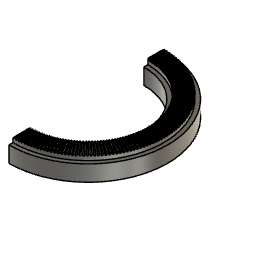
Angled Rack and BEVEL track system - Light output v2 (Autodesk Fusion 360 design; units mm, degrees)
Autodesk Fusion 360 part; units mm, degrees
sketch "Sketch1" plane through (0, 0, 0) normal (0, 0, 1) x (1, 0, 0)
  circle A0 centre (0, 0) radius 100
  dimension "d1" = 200
  constraint coincident A0.centre origin
  measures "d1" diameter of A0
sketch "Sketch2" plane through (0, 0, 0) normal (0, 0, 1) x (1, 0, 0)
  circle A0 centre (0, 0) radius 100
  line L0 (0, 100) -> (0, -100)
  constraint coincident A0 L0.start
  constraint coincident A0 L0.end
  constraint vertical L0
extrude "Extrude1" add sketch "Sketch2" along normal blind 20 contours A0 L0 picked at (53.8118, -17.5328)
sketch "Sketch3" plane through (0, 0, 20) normal (0, 0, 1) x (-1, 0, 0)
  line L0 (0, -100) -> (0, 100)
  arc A0 (0, 100) -> (0, -100) centre (0, 0) ccw
  circle A1 centre (0, 0) radius 70
  dimension "d4" = 140
  constraint coincident A0.centre A1.centre
  measures "d4" diameter of A1
extrude "Extrude2" cut sketch "Sketch3" against normal blind 30 contours L0 A1 picked at (-23.2681, 1.7437)
sketch "Sketch4" plane through (0, 0, 20) normal (0, 0, 1) x (-1, 0, 0)
  arc A0 (0, 70) -> (0, -70) centre (0, 0) ccw
  line L0 (0, 70) -> (0, 100)
  arc A1 (0, 100) -> (0, -100) centre (0, 0) ccw
  line L1 (0, -100) -> (0, -70)
  circle A2 centre (0, 0) radius 75
  circle A3 centre (0, 0) radius 95
  dimension "d7" = 150
  dimension "d8" = 190
  constraint coincident A0.centre A1.centre
  measures "d7" diameter of A2
  measures "d8" diameter of A3
extrude "Extrude3" add sketch "Sketch4" along normal blind 5 contours L0 L1 A2 A3 picked at (-4.7197, -87.9796)
sketch "Sketch5" plane through (0, 0, 25) normal (0, 0, 1) x (-1, 0, 0)
  line L0 (0, 75) -> (0, 95)
  arc A0 (0, 95) -> (0, -95) centre (0, 0) ccw
  line L1 (0, -95) -> (0, -75)
  arc A1 (0, 75) -> (0, -75) centre (0, 0) ccw
  line L2 (0, 0) -> (0, -95)
  line L3 (0, 0) -> (-1.658, -94.9855)
  line L4 (0, 0) -> (95, 0) construction
  line L5 (0, 0) -> (-3.3155, -94.9421)
  line L6 (0, 0) -> (95, 0) construction
  line L7 (0, 0) -> (-4.9719, -94.8698)
  line L8 (0, 0) -> (95, 0) construction
  line L9 (0, 0) -> (-6.6269, -94.7686)
  line L10 (0, 0) -> (95, 0) construction
  line L11 (0, 0) -> (-8.2798, -94.6385)
  line L12 (0, 0) -> (95, 0) construction
  line L13 (0, 0) -> (-9.9302, -94.4796)
  line L14 (0, 0) -> (95, 0) construction
  line L15 (0, 0) -> (-11.5776, -94.2919)
  line L16 (0, 0) -> (95, 0) construction
  line L17 (0, 0) -> (-13.2214, -94.0755)
  line L18 (0, 0) -> (95, 0) construction
  line L19 (0, 0) -> (-14.8613, -93.8304)
  line L20 (0, 0) -> (95, 0) construction
  line L21 (0, 0) -> (-16.4966, -93.5567)
  line L22 (0, 0) -> (95, 0) construction
  line L23 (0, 0) -> (-18.1269, -93.2546)
  line L24 (0, 0) -> (95, 0) construction
  line L25 (0, 0) -> (-19.7516, -92.924)
  line L26 (0, 0) -> (95, 0) construction
  line L27 (0, 0) -> (-21.3704, -92.5652)
  line L28 (0, 0) -> (95, 0) construction
  line L29 (0, 0) -> (-22.9826, -92.1781)
  line L30 (0, 0) -> (95, 0) construction
  line L31 (0, 0) -> (-24.5878, -91.763)
  line L32 (0, 0) -> (95, 0) construction
  line L33 (0, 0) -> (-26.1855, -91.3199)
  line L34 (0, 0) -> (95, 0) construction
  line L35 (0, 0) -> (-27.7753, -90.849)
  line L36 (0, 0) -> (95, 0) construction
  line L37 (0, 0) -> (-29.3566, -90.3504)
  line L38 (0, 0) -> (95, 0) construction
  line L39 (0, 0) -> (-30.929, -89.8243)
  line L40 (0, 0) -> (95, 0) construction
  line L41 (0, 0) -> (-32.4919, -89.2708)
  line L42 (0, 0) -> (95, 0) construction
  line L43 (0, 0) -> (-34.045, -88.6901)
  line L44 (0, 0) -> (95, 0) construction
  line L45 (0, 0) -> (-35.5876, -88.0825)
  line L46 (0, 0) -> (95, 0) construction
  line L47 (0, 0) -> (-37.1195, -87.448)
  line L48 (0, 0) -> (95, 0) construction
  line L49 (0, 0) -> (-38.64, -86.7868)
  line L50 (0, 0) -> (95, 0) construction
  line L51 (0, 0) -> (-40.1487, -86.0992)
  line L52 (0, 0) -> (95, 0) construction
  line L53 (0, 0) -> (-41.6453, -85.3854)
  line L54 (0, 0) -> (95, 0) construction
  line L55 (0, 0) -> (-43.1291, -84.6456)
  line L56 (0, 0) -> (95, 0) construction
  line L57 (0, 0) -> (-44.5998, -83.88)
  line L58 (0, 0) -> (95, 0) construction
  line L59 (0, 0) -> (-46.0569, -83.0889)
  line L60 (0, 0) -> (95, 0) construction
  line L61 (0, 0) -> (-47.5, -82.2724)
  line L62 (0, 0) -> (95, 0) construction
  line L63 (0, 0) -> (-48.9286, -81.4309)
  line L64 (0, 0) -> (95, 0) construction
  line L65 (0, 0) -> (-50.3423, -80.5646)
  line L66 (0, 0) -> (95, 0) construction
  line L67 (0, 0) -> (-51.7407, -79.6737)
  line L68 (0, 0) -> (95, 0) construction
  line L69 (0, 0) -> (-53.1233, -78.7586)
  line L70 (0, 0) -> (95, 0) construction
  line L71 (0, 0) -> (-54.4898, -77.8194)
  line L72 (0, 0) -> (95, 0) construction
  line L73 (0, 0) -> (-55.8396, -76.8566)
  line L74 (0, 0) -> (95, 0) construction
  line L75 (0, 0) -> (0, -2.1876)
  line L76 (0, 0) -> (-57.1724, -75.8704)
  line L77 (0, 0) -> (95, 0) construction
  line L78 (0, 0) -> (-58.4878, -74.861)
  line L79 (0, 0) -> (95, 0) construction
  line L80 (0, 0) -> (-59.7854, -73.8289)
  line L81 (0, 0) -> (95, 0) construction
  line L82 (0, 0) -> (-61.0648, -72.7742)
  line L83 (0, 0) -> (95, 0) construction
  line L84 (0, 0) -> (-62.3256, -71.6974)
  line L85 (0, 0) -> (95, 0) construction
  line L86 (0, 0) -> (-63.5674, -70.5988)
  line L87 (0, 0) -> (95, 0) construction
  line L88 (0, 0) -> (-64.7898, -69.4786)
  line L89 (0, 0) -> (95, 0) construction
  line L90 (0, 0) -> (-65.9925, -68.3373)
  line L91 (0, 0) -> (95, 0) construction
  line L92 (0, 0) -> (-67.1751, -67.1751)
  line L93 (0, 0) -> (95, 0) construction
  line L94 (0, 0) -> (-68.3373, -65.9925)
  line L95 (0, 0) -> (95, 0) construction
  line L96 (0, 0) -> (-69.4786, -64.7898)
  line L97 (0, 0) -> (95, 0) construction
  line L98 (0, 0) -> (-70.5988, -63.5674)
  line L99 (0, 0) -> (95, 0) construction
  line L100 (0, 0) -> (-71.6974, -62.3256)
  line L101 (0, 0) -> (95, 0) construction
  line L102 (0, 0) -> (-72.7742, -61.0648)
  line L103 (0, 0) -> (95, 0) construction
  line L104 (0, 0) -> (-73.8289, -59.7854)
  line L105 (0, 0) -> (95, 0) construction
  line L106 (0, 0) -> (-74.861, -58.4878)
  line L107 (0, 0) -> (95, 0) construction
  line L108 (0, 0) -> (-75.8704, -57.1724)
  line L109 (0, 0) -> (95, 0) construction
  line L110 (0, 0) -> (-76.8566, -55.8396)
  line L111 (0, 0) -> (95, 0) construction
  line L112 (0, 0) -> (-77.8194, -54.4898)
  line L113 (0, 0) -> (95, 0) construction
  line L114 (0, 0) -> (-78.7586, -53.1233)
  line L115 (0, 0) -> (95, 0) construction
  line L116 (0, 0) -> (-79.6737, -51.7407)
  line L117 (0, 0) -> (95, 0) construction
  line L118 (0, 0) -> (-80.5646, -50.3423)
  line L119 (0, 0) -> (95, 0) construction
  line L120 (0, 0) -> (-81.4309, -48.9286)
  line L121 (0, 0) -> (95, 0) construction
  line L122 (0, 0) -> (-82.2724, -47.5)
  line L123 (0, 0) -> (95, 0) construction
  line L124 (0, 0) -> (-83.0889, -46.0569)
  line L125 (0, 0) -> (95, 0) construction
  line L126 (0, 0) -> (-83.88, -44.5998)
  line L127 (0, 0) -> (95, 0) construction
  line L128 (0, 0) -> (-84.6456, -43.1291)
  line L129 (0, 0) -> (95, 0) construction
  line L130 (0, 0) -> (-85.3854, -41.6453)
  line L131 (0, 0) -> (95, 0) construction
  line L132 (0, 0) -> (94.9855, 0) construction
  line L133 (0, 0) -> (-86.7868, -38.64)
  line L134 (0, 0) -> (95, 0) construction
  line L135 (0, 0) -> (-87.448, -37.1195)
  line L136 (0, 0) -> (95, 0) construction
  line L137 (0, 0) -> (-88.0825, -35.5876)
  line L138 (0, 0) -> (95, 0) construction
  line L139 (0, 0) -> (-88.6901, -34.045)
  line L140 (0, 0) -> (95, 0) construction
  line L141 (0, 0) -> (-89.2708, -32.4919)
  line L142 (0, 0) -> (95, 0) construction
  line L143 (0, 0) -> (-89.8243, -30.929)
  line L144 (0, 0) -> (95, 0) construction
  line L145 (0, 0) -> (-90.3504, -29.3566)
  line L146 (0, 0) -> (95, 0) construction
  line L147 (0, 0) -> (-90.849, -27.7753)
  line L148 (0, 0) -> (95, 0) construction
  line L149 (0, 0) -> (-91.3199, -26.1855)
  line L150 (0, 0) -> (95, 0) construction
  line L151 (0, 0) -> (-91.763, -24.5878)
  line L152 (0, 0) -> (95, 0) construction
  line L153 (0, 0) -> (-92.1781, -22.9826)
  line L154 (0, 0) -> (95, 0) construction
  line L155 (0, 0) -> (-92.5652, -21.3704)
  line L156 (0, 0) -> (95, 0) construction
  line L157 (0, 0) -> (-92.924, -19.7516)
  line L158 (0, 0) -> (95, 0) construction
  line L159 (0, 0) -> (-93.2546, -18.1269)
  line L160 (0, 0) -> (95, 0) construction
  line L161 (0, 0) -> (-93.5567, -16.4966)
  line L162 (0, 0) -> (95, 0) construction
  line L163 (0, 0) -> (-93.8304, -14.8613)
  line L164 (0, 0) -> (95, 0) construction
  line L165 (0, 0) -> (-94.0755, -13.2214)
  line L166 (0, 0) -> (95, 0) construction
  line L167 (0, 0) -> (-94.2919, -11.5776)
  line L168 (0, 0) -> (95, 0) construction
  line L169 (0, 0) -> (-94.4796, -9.9302)
  line L170 (0, 0) -> (95, 0) construction
  line L171 (0, 0) -> (-94.6385, -8.2798)
  line L172 (0, 0) -> (95, 0) construction
  line L173 (0, 0) -> (-94.7686, -6.6269)
  line L174 (0, 0) -> (95, 0) construction
  line L175 (0, 0) -> (-94.8698, -4.9719)
  line L176 (0, 0) -> (95, 0) construction
  line L177 (0, 0) -> (-94.9421, -3.3155)
  line L178 (0, 0) -> (95, 0) construction
  line L179 (0, 0) -> (-94.9855, -1.658)
  line L180 (0, 0) -> (95, 0) construction
  line L181 (0, 0) -> (-95, 0)
  line L182 (0, 0) -> (-86.0992, -40.1487)
  line L183 (0, 0) -> (95, 0) construction
  dimension "d11" = 91
  dimension "d13" = 92
  dimension "d15" = 93
  dimension "d16" = 94
  dimension "d17" = 95
  dimension "d18" = 96
  dimension "d19" = 97
  dimension "d20" = 98
  dimension "d21" = 99
  dimension "d22" = 100
  dimension "d23" = 101
  dimension "d24" = 102
  dimension "d25" = 103
  dimension "d26" = 104
  dimension "d27" = 105
  dimension "d28" = 106
  dimension "d29" = 107
  dimension "d30" = 108
  dimension "d31" = 109
  dimension "d32" = 110
  dimension "d33" = 111
  dimension "d34" = 112
  dimension "d35" = 113
  dimension "d36" = 114
  dimension "d37" = 115
  dimension "d38" = 116
  dimension "d39" = 117
  dimension "d40" = 118
  dimension "d42" = 119
  dimension "d43" = 120
  dimension "d44" = 121
  dimension "d45" = 122
  dimension "d47" = 123
  dimension "d48" = 124
  dimension "d49" = 125
  dimension "d50" = 126
  dimension "d51" = 127
  dimension "d52" = 128
  dimension "d53" = 129
  dimension "d54" = 130
  dimension "d55" = 131
  dimension "d56" = 132
  dimension "d57" = 133
  dimension "d58" = 134
  dimension "d60" = 135
  dimension "d61" = 136
  dimension "d62" = 137
  dimension "d63" = 138
  dimension "d64" = 139
  dimension "d65" = 140
  dimension "d66" = 141
  dimension "d67" = 142
  dimension "d69" = 143
  dimension "d70" = 144
  dimension "d71" = 145
  dimension "d72" = 146
  dimension "d74" = 147
  dimension "d75" = 148
  dimension "d76" = 149
  dimension "d77" = 150
  dimension "d78" = 151
  dimension "d79" = 152
  dimension "d80" = 153
  dimension "d81" = 154
  dimension "d83" = 156
  dimension "d84" = 157
  dimension "d85" = 158
  dimension "d86" = 159
  dimension "d87" = 160
  dimension "d88" = 161
  dimension "d90" = 162
  dimension "d91" = 163
  dimension "d92" = 164
  dimension "d93" = 165
  dimension "d94" = 166
  dimension "d95" = 167
  dimension "d96" = 168
  dimension "d97" = 169
  dimension "d98" = 170
  dimension "d99" = 171
  dimension "d100" = 172
  dimension "d101" = 173
  dimension "d102" = 174
  dimension "d103" = 175
  dimension "d104" = 176
  dimension "d106" = 177
  dimension "d108" = 178
  dimension "d110" = 179
  dimension "d111" = 155
  constraint coincident A0.centre A1.centre
  constraint coincident A0.end L1.start
  constraint horizontal L4
  constraint horizontal L6
  constraint horizontal L8
  constraint horizontal L10
  constraint horizontal L12
  constraint horizontal L14
  constraint horizontal L16
  constraint horizontal L18
  constraint horizontal L20
  constraint horizontal L22
  constraint horizontal L24
  constraint horizontal L26
  constraint horizontal L28
  constraint horizontal L30
  constraint horizontal L32
  constraint horizontal L34
  constraint horizontal L36
  constraint horizontal L38
  constraint horizontal L40
  constraint horizontal L42
  constraint horizontal L44
  constraint horizontal L46
  constraint horizontal L48
  constraint horizontal L50
  constraint horizontal L52
  constraint horizontal L54
  constraint horizontal L56
  constraint horizontal L58
  constraint horizontal L60
  constraint horizontal L62
  constraint horizontal L64
  constraint horizontal L66
  constraint horizontal L68
  constraint horizontal L70
  constraint horizontal L72
  constraint horizontal L74
  constraint vertical L75
  constraint horizontal L77
  constraint horizontal L79
  constraint horizontal L81
  constraint horizontal L83
  constraint horizontal L85
  constraint horizontal L87
  constraint horizontal L89
  constraint horizontal L91
  constraint horizontal L93
  constraint horizontal L95
  constraint horizontal L97
  constraint horizontal L99
  constraint horizontal L101
  constraint horizontal L103
  constraint horizontal L105
  constraint horizontal L107
  constraint horizontal L109
  constraint horizontal L111
  constraint horizontal L113
  constraint horizontal L115
  constraint horizontal L117
  constraint horizontal L119
  constraint horizontal L121
  constraint horizontal L123
  constraint horizontal L125
  constraint horizontal L127
  constraint horizontal L129
  constraint horizontal L131
  constraint horizontal L132
  constraint horizontal L134
  constraint horizontal L136
  constraint horizontal L138
  constraint horizontal L140
  constraint horizontal L142
  constraint horizontal L144
  constraint horizontal L146
  constraint horizontal L148
  constraint horizontal L150
  constraint horizontal L152
  constraint horizontal L154
  constraint horizontal L156
  constraint horizontal L158
  constraint horizontal L160
  constraint horizontal L162
  constraint horizontal L164
  constraint horizontal L166
  constraint horizontal L168
  constraint horizontal L170
  constraint horizontal L172
  constraint horizontal L174
  constraint horizontal L176
  constraint horizontal L178
  constraint horizontal L180
  constraint midpoint A0 L181.end
  constraint horizontal L183
  measures "d11" angle of L3 L4
  measures "d13" angle of L5 L6
  measures "d15" angle of L7 L8
  measures "d16" angle of L9 L10
  measures "d17" angle of L11 L12
  measures "d18" angle of L13 L14
  measures "d19" angle of L15 L16
  measures "d20" angle of L17 L18
  measures "d21" angle of L19 L20
  measures "d22" angle of L21 L22
  measures "d23" angle of L23 L24
  measures "d24" angle of L25 L26
  measures "d25" angle of L27 L28
  measures "d26" angle of L29 L30
  measures "d27" angle of L31 L32
  measures "d28" angle of L33 L34
  measures "d29" angle of L35 L36
  measures "d30" angle of L37 L38
  measures "d31" angle of L39 L40
  measures "d32" angle of L41 L42
  measures "d33" angle of L43 L44
  measures "d34" angle of L45 L46
  measures "d35" angle of L47 L48
  measures "d36" angle of L49 L50
  measures "d37" angle of L51 L52
  measures "d38" angle of L53 L54
  measures "d39" angle of L55 L56
  measures "d40" angle of L57 L58
  measures "d42" angle of L59 L60
  measures "d43" angle of L61 L62
  measures "d44" angle of L63 L64
  measures "d45" angle of L65 L66
  measures "d47" angle of L67 L68
  measures "d48" angle of L69 L70
  measures "d49" angle of L71 L72
  measures "d50" angle of L73 L74
  measures "d51" angle of L76 L77
  measures "d52" angle of L78 L79
  measures "d53" angle of L80 L81
  measures "d54" angle of L82 L83
  measures "d55" angle of L84 L85
  measures "d56" angle of L86 L87
  measures "d57" angle of L88 L89
  measures "d58" angle of L90 L91
  measures "d60" angle of L92 L93
  measures "d61" angle of L94 L95
  measures "d62" angle of L96 L97
  measures "d63" angle of L98 L99
  measures "d64" angle of L100 L101
  measures "d65" angle of L102 L103
  measures "d66" angle of L104 L105
  measures "d67" angle of L106 L107
  measures "d69" angle of L108 L109
  measures "d70" angle of L110 L111
  measures "d71" angle of L112 L113
  measures "d72" angle of L114 L115
  measures "d74" angle of L116 L117
  measures "d75" angle of L118 L119
  measures "d76" angle of L120 L121
  measures "d77" angle of L122 L123
  measures "d78" angle of L124 L125
  measures "d79" angle of L126 L127
  measures "d80" angle of L128 L129
  measures "d81" angle of L130 L131
  measures "d83" angle of L133 L134
  measures "d84" angle of L135 L136
  measures "d85" angle of L137 L138
  measures "d86" angle of L139 L140
  measures "d87" angle of L141 L142
  measures "d88" angle of L143 L144
  measures "d90" angle of L145 L146
  measures "d91" angle of L147 L148
  measures "d92" angle of L149 L150
  measures "d93" angle of L151 L152
  measures "d94" angle of L153 L154
  measures "d95" angle of L155 L156
  measures "d96" angle of L157 L158
  measures "d97" angle of L159 L160
  measures "d98" angle of L161 L162
  measures "d99" angle of L163 L164
  measures "d100" angle of L165 L166
  measures "d101" angle of L167 L168
  measures "d102" angle of L169 L170
  measures "d103" angle of L171 L172
  measures "d104" angle of L173 L174
  measures "d106" angle of L175 L176
  measures "d108" angle of L177 L178
  measures "d110" angle of L179 L180
  measures "d111" angle of L182 L183
sketch "Sketch6" plane through (0, 0, 25) normal (0, 0, 1) x (-1, 0, 0)
sketch "Sketch7" plane through (0, 0, 25) normal (0, 0, 1) x (-1, 0, 0)
sketch "Sketch8" plane through (0, 0, 25) normal (0, 0, 1) x (-1, 0, 0)
extrude "Extrude4" add sketch "Sketch5" along normal blind 2 contours A0 A1 L177 L179 | A0 L1 A1 L2 L3 | A0 A1 L5 L7 | A0 A1 L9 L11 | A0 A1 L13 L15 | A0 A1 L17 L19 | A0 A1 L21 L23 | A0 A1 L25 L27 | A0 A1 L29 L31 | A0 A1 L33 L35 | A0 A1 L37 L39 | A0 A1 L41 L43 | A0 A1 L45 L47 | A0 A1 L49 L51 | A0 A1 L53 L55 | A0 A1 L57 L59 | A0 A1 L61 L63 | A0 A1 L65 L67 | A0 A1 L69 L71 | A0 A1 L73 L76 | A0 A1 L78 L80 | A0 A1 L82 L84 | A0 A1 L86 L88 | A0 A1 L90 L92 | A0 A1 L94 L96 | A0 A1 L98 L100 | A0 A1 L102 L104 | A0 A1 L106 L108 | A0 A1 L110 L112 | A0 A1 L114 L116 | A0 A1 L118 L120 | A0 A1 L122 L124 | A0 A1 L126 L128 | A0 A1 L130 L182 | A0 A1 L133 L135 | A0 A1 L137 L139 | A0 A1 L141 L143 | A0 A1 L145 L147 | A0 A1 L149 L151 | A0 A1 L153 L155 | A0 A1 L157 L159 | A0 A1 L161 L163 | A0 A1 L165 L167 | A0 A1 L169 L171 | A0 A1 L173 L175
sketch "Sketch9" plane through (0, 0, 25) normal (0, 0, 1) x (-1, 0, 0)
  line L0 (-94.9855, -1.658) -> (-74.9886, -1.3089)
  arc A0 (0, 75) -> (-74.9886, -1.3089) centre (0, 0) ccw
  line L1 (0, 75) -> (0, 95)
  arc A1 (0, 95) -> (-94.9855, -1.658) centre (0, 0) ccw
  line L2 (0, 0) -> (-95, 0)
  line L3 (0, 0) -> (-94.9855, 1.658)
  line L4 (0, 0) -> (95, 0) construction
  line L5 (0, 0) -> (-94.9421, 3.3155)
  line L6 (0, 0) -> (95, 0) construction
  line L7 (0, 0) -> (-94.8698, 4.9719)
  line L8 (0, 0) -> (95, 0) construction
  line L9 (0, 0) -> (94.9855, 0) construction
  line L10 (0, 0) -> (94.9855, 0) construction
  line L11 (0, 0) -> (-94.4796, 9.9302)
  line L12 (0, 0) -> (95, 0) construction
  line L13 (0, 0) -> (-94.2919, 11.5776)
  line L14 (0, 0) -> (95, 0) construction
  line L15 (0, 0) -> (-94.0755, 13.2214)
  line L16 (0, 0) -> (94.9421, 0) construction
  line L17 (0, 0) -> (-93.8304, 14.8613)
  line L18 (0, 0) -> (95, 0) construction
  line L19 (0, 0) -> (-93.5567, 16.4966)
  line L20 (0, 0) -> (95, 0) construction
  line L21 (0, 0) -> (-93.2546, 18.1269)
  line L22 (0, 0) -> (95, 0) construction
  line L23 (0, 0) -> (-92.924, 19.7516)
  line L24 (0, 0) -> (95, 0) construction
  line L25 (0, 0) -> (-92.5652, 21.3704)
  line L26 (0, 0) -> (95, 0) construction
  line L27 (0, 0) -> (-92.1781, 22.9826)
  line L28 (0, 0) -> (95, 0) construction
  line L29 (0, 0) -> (-91.763, 24.5878)
  line L30 (0, 0) -> (95, 0) construction
  line L31 (0, 0) -> (-91.3199, 26.1855)
  line L32 (0, 0) -> (95, 0) construction
  line L33 (0, 0) -> (-90.849, 27.7753)
  line L34 (0, 0) -> (95, 0) construction
  line L35 (0, 0) -> (-90.3504, 29.3566)
  line L36 (0, 0) -> (95, 0) construction
  line L37 (0, 0) -> (-89.8243, 30.929)
  line L38 (0, 0) -> (95, 0) construction
  line L39 (0, 0) -> (-89.2708, 32.4919)
  line L40 (0, 0) -> (95, 0) construction
  line L41 (0, 0) -> (-88.6901, 34.045)
  line L42 (0, 0) -> (95, 0) construction
  line L43 (0, 0) -> (-88.0825, 35.5876)
  line L44 (0, 0) -> (95, 0) construction
  line L45 (0, 0) -> (-87.448, 37.1195)
  line L46 (0, 0) -> (95, 0) construction
  line L47 (0, 0) -> (-86.7868, 38.64)
  line L48 (0, 0) -> (95, 0) construction
  line L49 (0, 0) -> (-86.0992, 40.1487)
  line L50 (0, 0) -> (95, 0) construction
  line L51 (0, 0) -> (-85.3854, 41.6453)
  line L52 (0, 0) -> (95, 0) construction
  line L53 (0, 0) -> (-84.6456, 43.1291)
  line L54 (0, 0) -> (95, 0) construction
  line L55 (0, 0) -> (-83.88, 44.5998)
  line L56 (0, 0) -> (95, 0) construction
  line L57 (0, 0) -> (-83.0889, 46.0569)
  line L58 (0, 0) -> (95, 0) construction
  line L59 (0, 0) -> (-82.2724, 47.5)
  line L60 (0, 0) -> (95, 0) construction
  line L61 (0, 0) -> (-81.4309, 48.9286)
  line L62 (0, 0) -> (95, 0) construction
  line L63 (0, 0) -> (-80.5646, 50.3423)
  line L64 (0, 0) -> (95, 0) construction
  line L65 (0, 0) -> (-79.6737, 51.7407)
  line L66 (0, 0) -> (95, 0) construction
  line L67 (0, 0) -> (-78.7586, 53.1233)
  line L68 (0, 0) -> (95, 0) construction
  line L69 (0, 0) -> (-77.8194, 54.4898)
  line L70 (0, 0) -> (95, 0) construction
  line L71 (0, 0) -> (-76.8566, 55.8396)
  line L72 (0, 0) -> (95, 0) construction
  line L73 (0, 0) -> (-75.8704, 57.1724)
  line L74 (0, 0) -> (95, 0) construction
  line L75 (0, 0) -> (-74.861, 58.4878)
  line L76 (0, 0) -> (95, 0) construction
  line L77 (0, 0) -> (-73.8289, 59.7854)
  line L78 (0, 0) -> (95, 0) construction
  line L79 (0, 0) -> (-72.7742, 61.0648)
  line L80 (0, 0) -> (95, 0) construction
  line L81 (0, 0) -> (-71.6974, 62.3256)
  line L82 (0, 0) -> (95, 0) construction
  line L83 (0, 0) -> (-70.5988, 63.5674)
  line L84 (0, 0) -> (95, 0) construction
  line L85 (0, 0) -> (94.9855, 0) construction
  line L86 (0, 0) -> (-68.3373, 65.9925)
  line L87 (0, 0) -> (95, 0) construction
  line L88 (0, 0) -> (-67.1751, 67.1751)
  line L89 (0, 0) -> (95, 0) construction
  line L90 (0, 0) -> (-65.9925, 68.3373)
  line L91 (0, 0) -> (95, 0) construction
  line L92 (0, 0) -> (-64.7898, 69.4786)
  line L93 (0, 0) -> (95, 0) construction
  line L94 (0, 0) -> (-63.5674, 70.5988)
  line L95 (0, 0) -> (95, 0) construction
  line L96 (0, 0) -> (-62.3256, 71.6974)
  line L97 (0, 0) -> (95, 0) construction
  line L98 (0, 0) -> (-61.0648, 72.7742)
  line L99 (0, 0) -> (95, 0) construction
  line L100 (0, 0) -> (94.9855, 0) construction
  line L101 (0, 0) -> (-58.4878, 74.861)
  line L102 (0, 0) -> (95, 0) construction
  line L103 (0, 0) -> (-57.1724, 75.8704)
  line L104 (0, 0) -> (95, 0) construction
  line L105 (0, 0) -> (-55.8396, 76.8566)
  line L106 (0, 0) -> (95, 0) construction
  line L107 (0, 0) -> (-54.4898, 77.8194)
  line L108 (0, 0) -> (95, 0) construction
  line L109 (0, 0) -> (-53.1233, 78.7586)
  line L110 (0, 0) -> (95, 0) construction
  line L111 (0, 0) -> (-51.7407, 79.6737)
  line L112 (0, 0) -> (95, 0) construction
  line L113 (0, 0) -> (-50.3423, 80.5646)
  line L114 (0, 0) -> (95, 0) construction
  line L115 (0, 0) -> (-48.9286, 81.4309)
  line L116 (0, 0) -> (95, 0) construction
  line L117 (0, 0) -> (-47.5, 82.2724)
  line L118 (0, 0) -> (95, 0) construction
  line L119 (0, 0) -> (-46.0569, 83.0889)
  line L120 (0, 0) -> (95, 0) construction
  line L121 (0, 0) -> (-44.5998, 83.88)
  line L122 (0, 0) -> (95, 0) construction
  line L123 (0, 0) -> (-43.1291, 84.6456)
  line L124 (0, 0) -> (95, 0) construction
  line L125 (0, 0) -> (-41.6453, 85.3854)
  line L126 (0, 0) -> (95, 0) construction
  line L127 (0, 0) -> (-40.1487, 86.0992)
  line L128 (0, 0) -> (95, 0) construction
  line L129 (0, 0) -> (-38.64, 86.7868)
  line L130 (0, 0) -> (95, 0) construction
  line L131 (0, 0) -> (-37.1195, 87.448)
  line L132 (0, 0) -> (95, 0) construction
  line L133 (0, 0) -> (-35.5876, 88.0825)
  line L134 (0, 0) -> (95, 0) construction
  line L135 (0, 0) -> (-34.045, 88.6901)
  line L136 (0, 0) -> (95, 0) construction
  line L137 (0, 0) -> (-32.4919, 89.2708)
  line L138 (0, 0) -> (95, 0) construction
  line L139 (0, 0) -> (-30.929, 89.8243)
  line L140 (0, 0) -> (95, 0) construction
  line L141 (0, 0) -> (-29.3566, 90.3504)
  line L142 (0, 0) -> (95, 0) construction
  line L143 (0, 0) -> (-27.7753, 90.849)
  line L144 (0, 0) -> (95, 0) construction
  line L145 (0, 0) -> (-26.1855, 91.3199)
  line L146 (0, 0) -> (95, 0) construction
  line L147 (0, 0) -> (-24.5878, 91.763)
  line L148 (0, 0) -> (95, 0) construction
  line L149 (0, 0) -> (-22.9826, 92.1781)
  line L150 (0, 0) -> (95, 0) construction
  line L151 (0, 0) -> (-21.3704, 92.5652)
  line L152 (0, 0) -> (95, 0) construction
  line L153 (0, 0) -> (-19.7516, 92.924)
  line L154 (0, 0) -> (95, 0) construction
  line L155 (0, 0) -> (-18.1269, 93.2546)
  line L156 (0, 0) -> (95, 0) construction
  line L157 (0, 0) -> (-16.4966, 93.5567)
  line L158 (0, 0) -> (95, 0) construction
  line L159 (0, 0) -> (-14.8613, 93.8304)
  line L160 (0, 0) -> (95, 0) construction
  line L161 (0, 0) -> (-13.2214, 94.0755)
  line L162 (0, 0) -> (95, 0) construction
  line L163 (0, 0) -> (-11.5776, 94.2919)
  line L164 (0, 0) -> (95, 0) construction
  line L165 (0, 0) -> (-9.9302, 94.4796)
  line L166 (0, 0) -> (95, 0) construction
  line L167 (0, 0) -> (-8.2798, 94.6385)
  line L168 (0, 0) -> (95, 0) construction
  line L169 (0, 0) -> (-6.6269, 94.7686)
  line L170 (0, 0) -> (95, 0) construction
  line L171 (0, 0) -> (-4.9719, 94.8698)
  line L172 (0, 0) -> (95, 0) construction
  line L173 (0, 0) -> (-3.3155, 94.9421)
  line L174 (0, 0) -> (95, 0) construction
  line L175 (0, 0) -> (94.9855, 0) construction
  line L176 (0, 0) -> (0, 95)
  line L177 (0, 0) -> (-94.7686, 6.6269)
  line L178 (0, 0) -> (95, 0) construction
  line L179 (0, 0) -> (-94.6385, 8.2798)
  line L180 (0, 0) -> (94.9855, 0) construction
  line L181 (0, 0) -> (-69.4786, 64.7898)
  line L182 (0, 0) -> (95, 0) construction
  line L183 (0, 0) -> (-59.7854, 73.8289)
  line L184 (0, 0) -> (95, 0) construction
  line L185 (0, 0) -> (-1.658, 94.9855)
  line L186 (0, 0) -> (95, 0) construction
  dimension "d114" = 179
  dimension "d116" = 178
  dimension "d117" = 177
  dimension "d120" = 174
  dimension "d122" = 173
  dimension "d123" = 172
  dimension "d125" = 171
  dimension "d126" = 170
  dimension "d127" = 169
  dimension "d128" = 168
  dimension "d129" = 167
  dimension "d130" = 166
  dimension "d131" = 165
  dimension "d132" = 164
  dimension "d133" = 163
  dimension "d134" = 162
  dimension "d135" = 161
  dimension "d136" = 160
  dimension "d137" = 159
  dimension "d138" = 158
  dimension "d139" = 157
  dimension "d140" = 156
  dimension "d141" = 155
  dimension "d142" = 154
  dimension "d143" = 153
  dimension "d144" = 152
  dimension "d145" = 151
  dimension "d146" = 150
  dimension "d147" = 149
  dimension "d148" = 148
  dimension "d149" = 147
  dimension "d150" = 146
  dimension "d151" = 145
  dimension "d152" = 144
  dimension "d153" = 143
  dimension "d154" = 142
  dimension "d155" = 141
  dimension "d156" = 140
  dimension "d157" = 139
  dimension "d158" = 138
  dimension "d160" = 136
  dimension "d161" = 135
  dimension "d162" = 134
  dimension "d163" = 133
  dimension "d164" = 132
  dimension "d166" = 131
  dimension "d167" = 130
  dimension "d169" = 128
  dimension "d170" = 127
  dimension "d171" = 126
  dimension "d172" = 125
  dimension "d173" = 124
  dimension "d174" = 123
  dimension "d175" = 122
  dimension "d176" = 121
  dimension "d177" = 120
  dimension "d178" = 119
  dimension "d179" = 118
  dimension "d180" = 117
  dimension "d181" = 116
  dimension "d182" = 115
  dimension "d183" = 114
  dimension "d184" = 113
  dimension "d185" = 112
  dimension "d186" = 111
  dimension "d188" = 110
  dimension "d189" = 109
  dimension "d190" = 108
  dimension "d191" = 107
  dimension "d193" = 106
  dimension "d195" = 105
  dimension "d196" = 104
  dimension "d197" = 103
  dimension "d198" = 102
  dimension "d199" = 101
  dimension "d201" = 100
  dimension "d202" = 99
  dimension "d204" = 98
  dimension "d205" = 97
  dimension "d206" = 96
  dimension "d207" = 95
  dimension "d209" = 94
  dimension "d210" = 93
  dimension "d211" = 92
  dimension "d214" = 176
  dimension "d216" = 175
  dimension "d218" = 137
  dimension "d219" = 129
  dimension "d220" = 91
  constraint coincident A0.centre A1.centre
  constraint coincident A1 L2.end
  constraint horizontal L2
  constraint horizontal L4
  constraint horizontal L6
  constraint horizontal L8
  constraint horizontal L9
  constraint horizontal L10
  constraint horizontal L12
  constraint horizontal L14
  constraint horizontal L16
  constraint horizontal L18
  constraint horizontal L20
  constraint horizontal L22
  constraint horizontal L24
  constraint horizontal L26
  constraint horizontal L28
  constraint horizontal L30
  constraint horizontal L32
  constraint horizontal L34
  constraint horizontal L36
  constraint horizontal L38
  constraint coincident A1 L37.end
  constraint horizontal L40
  constraint horizontal L42
  constraint horizontal L44
  constraint horizontal L46
  constraint horizontal L48
  constraint horizontal L50
  constraint horizontal L52
  constraint horizontal L54
  constraint horizontal L56
  constraint horizontal L58
  constraint horizontal L60
  constraint horizontal L62
  constraint horizontal L64
  constraint horizontal L66
  constraint horizontal L68
  constraint coincident A1 L67.end
  constraint horizontal L70
  constraint horizontal L72
  constraint horizontal L74
  constraint horizontal L76
  constraint horizontal L78
  constraint horizontal L80
  constraint horizontal L82
  constraint horizontal L84
  constraint horizontal L85
  constraint horizontal L87
  constraint horizontal L89
  constraint horizontal L91
  constraint horizontal L93
  constraint horizontal L95
  constraint horizontal L97
  constraint horizontal L99
  constraint horizontal L100
  constraint horizontal L102
  constraint horizontal L104
  constraint horizontal L106
  constraint horizontal L108
  constraint horizontal L110
  constraint horizontal L112
  constraint horizontal L114
  constraint horizontal L116
  constraint horizontal L118
  constraint horizontal L120
  constraint horizontal L122
  constraint horizontal L124
  constraint horizontal L126
  constraint horizontal L128
  constraint horizontal L130
  constraint horizontal L132
  constraint horizontal L134
  constraint horizontal L136
  constraint horizontal L138
  constraint horizontal L140
  constraint horizontal L142
  constraint horizontal L144
  constraint horizontal L146
  constraint horizontal L148
  constraint horizontal L150
  constraint horizontal L152
  constraint horizontal L154
  constraint horizontal L156
  constraint horizontal L158
  constraint horizontal L160
  constraint horizontal L162
  constraint horizontal L164
  constraint horizontal L166
  constraint horizontal L168
  constraint horizontal L170
  constraint horizontal L172
  constraint horizontal L174
  constraint horizontal L175
  constraint coincident L1.end A1.start
  constraint horizontal L178
  constraint horizontal L180
  constraint horizontal L182
  constraint horizontal L184
  constraint horizontal L186
  measures "d114" angle of L3 L4
  measures "d116" angle of L5 L6
  measures "d117" angle of L7 L8
  measures "d120" angle of L11 L12
  measures "d122" angle of L13 L14
  measures "d123" angle of L15 L16
  measures "d125" angle of L17 L18
  measures "d126" angle of L19 L20
  measures "d127" angle of L21 L22
  measures "d128" angle of L23 L24
  measures "d129" angle of L25 L26
  measures "d130" angle of L27 L28
  measures "d131" angle of L29 L30
  measures "d132" angle of L31 L32
  measures "d133" angle of L33 L34
  measures "d134" angle of L35 L36
  measures "d135" angle of L37 L38
  measures "d136" angle of L39 L40
  measures "d137" angle of L41 L42
  measures "d138" angle of L43 L44
  measures "d139" angle of L45 L46
  measures "d140" angle of L47 L48
  measures "d141" angle of L49 L50
  measures "d142" angle of L51 L52
  measures "d143" angle of L53 L54
  measures "d144" angle of L55 L56
  measures "d145" angle of L57 L58
  measures "d146" angle of L59 L60
  measures "d147" angle of L61 L62
  measures "d148" angle of L63 L64
  measures "d149" angle of L65 L66
  measures "d150" angle of L67 L68
  measures "d151" angle of L69 L70
  measures "d152" angle of L71 L72
  measures "d153" angle of L73 L74
  measures "d154" angle of L75 L76
  measures "d155" angle of L77 L78
  measures "d156" angle of L79 L80
  measures "d157" angle of L81 L82
  measures "d158" angle of L83 L84
  measures "d160" angle of L86 L87
  measures "d161" angle of L88 L89
  measures "d162" angle of L90 L91
  measures "d163" angle of L92 L93
  measures "d164" angle of L94 L95
  measures "d166" angle of L96 L97
  measures "d167" angle of L98 L99
  measures "d169" angle of L101 L102
  measures "d170" angle of L103 L104
  measures "d171" angle of L105 L106
  measures "d172" angle of L107 L108
  measures "d173" angle of L109 L110
  measures "d174" angle of L111 L112
  measures "d175" angle of L113 L114
  measures "d176" angle of L115 L116
  measures "d177" angle of L117 L118
  measures "d178" angle of L119 L120
  measures "d179" angle of L121 L122
  measures "d180" angle of L123 L124
  measures "d181" angle of L125 L126
  measures "d182" angle of L127 L128
  measures "d183" angle of L129 L130
  measures "d184" angle of L131 L132
  measures "d185" angle of L133 L134
  measures "d186" angle of L135 L136
  measures "d188" angle of L137 L138
  measures "d189" angle of L139 L140
  measures "d190" angle of L141 L142
  measures "d191" angle of L143 L144
  measures "d193" angle of L145 L146
  measures "d195" angle of L147 L148
  measures "d196" angle of L149 L150
  measures "d197" angle of L151 L152
  measures "d198" angle of L153 L154
  measures "d199" angle of L155 L156
  measures "d201" angle of L157 L158
  measures "d202" angle of L159 L160
  measures "d204" angle of L161 L162
  measures "d205" angle of L163 L164
  measures "d206" angle of L165 L166
  measures "d207" angle of L167 L168
  measures "d209" angle of L169 L170
  measures "d210" angle of L171 L172
  measures "d211" angle of L173 L174
  measures "d214" angle of L177 L178
  measures "d216" angle of L179 L180
  measures "d218" angle of L181 L182
  measures "d219" angle of L183 L184
  measures "d220" angle of L185 L186
sketch "Sketch10" plane through (0, 0, 25) normal (0, 0, 1) x (-1, 0, 0)
sketch "Sketch11" plane through (0, 0, 25) normal (0, 0, 1) x (-1, 0, 0)
extrude "Extrude5" add sketch "Sketch9" along normal blind 2 contours A0 A1 L2 L3 | A0 A1 L5 L7 | A0 A1 L11 L13 | A0 A1 L15 L17 | A0 A1 L19 L21 | A0 A1 L23 L25 | A0 A1 L27 L29 | A0 A1 L31 L33 | A0 A1 L35 L37 | A0 A1 L39 L41 | A0 A1 L43 L45 | A0 A1 L47 L49 | A0 A1 L51 L53 | A0 A1 L55 L57 | A0 A1 L59 L61 | A0 A1 L63 L65 | A0 A1 L67 L69 | A0 A1 L71 L73 | A0 A1 L75 L77 | A0 A1 L79 L81 | A0 A1 L83 L181 | A0 A1 L86 L88 | A0 A1 L90 L92 | A0 A1 L94 L96 | A0 A1 L98 L183 | A0 A1 L101 L103 | A0 A1 L105 L107 | A0 A1 L109 L111 | A0 A1 L113 L115 | A0 A1 L117 L119 | A0 A1 L121 L123 | A0 A1 L125 L127 | A0 A1 L129 L131 | A0 A1 L133 L135 | A0 A1 L137 L139 | A0 A1 L141 L143 | A0 A1 L145 L147 | A0 A1 L149 L151 | A0 A1 L153 L155 | A0 A1 L157 L159 | A0 A1 L161 L163 | A0 A1 L165 L167 | A0 A1 L169 L171 | A0 A1 L173 L185 | A0 A1 L177 L179
